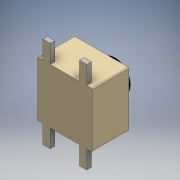
# Autodesk Inventor part: Touch Button
Saved by Autodesk Inventor 2016 SP1 (Build 200210100, 210)
## iProperties
Created: 2018-06-08
Part Number: Touch Button
Material: Générique
Document SubType Name: Modeling
Designer: dimercur
Density: 1 g/cm^3
Appearance: Par défaut
Author: dimercur
Autodesk Inventor part; units mm, degrees
ref_plane "YZ Plane" through (0, 0, 0) normal (1, 0, 0) x (0, 1, 0)
ref_plane "XZ Plane" through (0, 0, 0) normal (0, 1, 0) x (-1, 0, 0)
ref_plane "XY Plane" through (0, 0, 0) normal (0, 0, 1) x (1, 0, 0)
sketch "Esquisse1" plane through (0, 0, 0) normal (0, 1, 0) x (-1, 0, 0)
  line L0 (3, -3) -> (-3, -3)
  line L1 (-3, -3) -> (-3, 3)
  line L2 (-3, 3) -> (3, 3)
  line L3 (3, 3) -> (3, -3)
  point P0 (0, 0)
  dimension "d0" = 3
  dimension "d1" = 6
  dimension "d2" = 6
  dimension "d3" = 3
  constraints: 8 end point, 2 parallel, 2 perpendicular, 1 horizontal
  measures "d0" horizontal distance of point (0, 0) L0.start
  measures "d1" distance of L0.start L0.end
  measures "d2" distance of L2.end L0.start
  measures "d3" horizontal distance of point (0, 0) L0.start
extrude "Extrusion1" add sketch "Esquisse1" along normal blind 4
sketch "Esquisse2" plane through (0, 4, 0) normal (0, 1, 0) x (1, 0, 0)
  circle A0 centre (0, 0) radius 1.75
  dimension "d6" = 3.5
  constraints: 1 centre point, 1 coincident
  measures "d6" diameter of A0
extrude "Extrusion2" add sketch "Esquisse2" along normal blind 1.5
sketch "Esquisse3" plane through (0, 4, 0) normal (0, 1, 0) x (1, 0, 0)
  circle A0 centre (-2.2, -2.2) radius 0.6
  line L0 (-3, -3) -> (3, -3) projected
  line L1 (-3, 3) -> (-3, -3) projected
  circle A1 centre (2.2, -2.2) radius 0.6
  circle A2 centre (-2.2, 2.2) radius 0.6
  circle A3 centre (2.2, 2.2) radius 0.6
  point P0 (0, 0)
  dimension "d9" = 0.8
  dimension "d10" = 0.8
  dimension "d11" = 1.2
  dimension "d14" = 4.4
  dimension "d17" = 4.4
  constraints: 4 centre point, 1 horizontal, 1 vertical, 6 other
  measures "d9" distance from line of L0 A0.centre
  measures "d10" distance from line of L1 A0.centre
  measures "d11" diameter of A0
  measures "d14" distance of A0.centre A1.centre
  measures "d17" distance of A0.centre A2.centre
extrude "Extrusion3" add sketch "Esquisse3" along normal blind 0.4
sketch "Esquisse4" plane through (0, 0, 0) normal (0, -1, 0) x (1, 0, 0)
  line L0 (-3, 3) -> (3, 3) projected
  line L1 (2.4, 3) -> (1.6, 3)
  line L2 (1.6, 3) -> (1.6, 5)
  line L3 (1.6, 5) -> (2.4, 5)
  line L4 (2.4, 5) -> (2.4, 3)
  line L5 (3, -3) -> (3, 3) projected
  line L6 (2.4, -5) -> (1.6, -5)
  line L7 (1.6, -5) -> (1.6, -3)
  line L8 (1.6, -3) -> (2.4, -3)
  line L9 (2.4, -3) -> (2.4, -5)
  line L10 (-1.6, 3) -> (-2.4, 3)
  line L11 (-2.4, 3) -> (-2.4, 5)
  line L12 (-2.4, 5) -> (-1.6, 5)
  line L13 (-1.6, 5) -> (-1.6, 3)
  line L14 (-1.6, -5) -> (-2.4, -5)
  line L15 (-2.4, -5) -> (-2.4, -3)
  line L16 (-2.4, -3) -> (-1.6, -3)
  line L17 (-1.6, -3) -> (-1.6, -5)
  point P0 (0, 0)
  dimension "d22" = 2
  dimension "d23" = 0.8
  dimension "d24" = 0.6
  dimension "d27" = 8
  dimension "d30" = 4
  constraints: 32 end point, 2 horizontal, 2 parallel, 1 perpendicular, 1 point on line, 1 vertical, 24 other
  measures "d22" distance of L3.end L1.start
  measures "d23" distance of L2.end L3.end
  measures "d24" distance between parallel lines of L5 L4
  measures "d27" distance of L1.start L6.start
  measures "d30" distance of L1.start L10.start
extrude "Extrusion4" add sketch "Esquisse4" against normal blind 0.5
fillet "Congé1" radius 0.5 4 edges at (1.6, 4.4, 2.2) (-2.8, 4.4, 2.2) (-2.8, 4.4, -2.2) (1.6, 4.4, -2.2)
fillet "Congé2" radius 0.1 1 edges at (-1.75, 5.5, 0)
fillet "Congé3" radius 0.1 4 edges at (3, 2, 3) (3, 2, -3) (-3, 2, -3) (-3, 2, 3)
equation "\"d0\" = 0.5 * d1"
equation "\"d3\" = 0.5 * d2"
equation "\"d10\" = d9"
